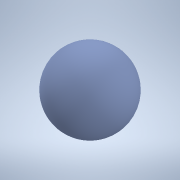
# Autodesk Inventor part: ball
Saved by Autodesk Inventor 2020 (Build 240168000, 168)
## iProperties
Created: 2020-06-27
Part Number: ball
Material: ゴム
Document SubType Name: Modeling
Designer: haya
Density: 0.93 g/cm^3
Appearance: ゴム - 青
Author: haya
Autodesk Inventor part; units mm, degrees
ref_plane "YZ Plane" through (0, 0, 0) normal (1, 0, 0) x (0, 1, 0)
ref_plane "XZ Plane" through (0, 0, 0) normal (0, 1, 0) x (-1, 0, 0)
ref_plane "XY Plane" through (0, 0, 0) normal (0, 0, 1) x (1, 0, 0)
sketch "スケッチ1" plane through (0, 0, 0) normal (0, 0, 1) x (1, 0, 0)
  arc A0 (0, -32.5) -> (0, 32.5) centre (0, 0) ccw
  line L0 (0, 0) -> (0, 32.5)
  line L1 (0, 0) -> (0, -32.5)
  dimension "d0" = 65
  constraints: 4 end point, 2 point on circle, 1 centre point, 1 coincident, 1 point on line, 1 vertical
  measures "d0" diameter of A0
revolve "回転1" add sketch "スケッチ1" angle 360 about axis through (0, 0, 0) along (0, 1, 0)
